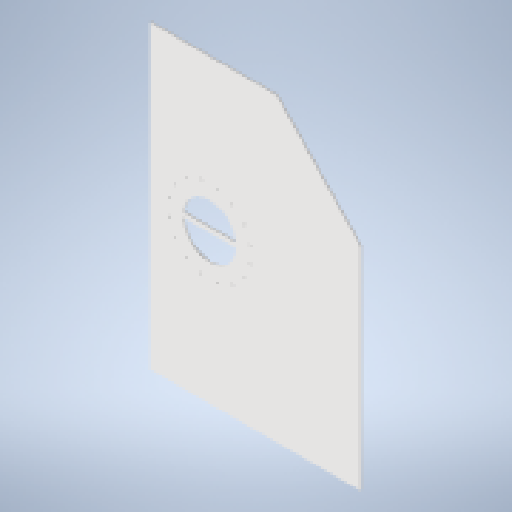
# Autodesk Inventor part: ДМФ 012 Стенка Корма ПРАВ
Saved by Autodesk Inventor 2024.2 (Build 282272000, 272)
## iProperties
Created: 2023-08-31
Part Number: ДМФ 012 Стенка Корма ПРАВ
Material: Generic
Document SubType Name: Sheet Metal
Designer: admin
Stock Number: ДМФ 010 Стенка_Корма
Density: 1 g/cm^3
Flat Pattern Width: 134 cm
Flat Pattern Length: 191 cm
Flat Pattern Area: 25594 cm^2
Sheet Metal Rule: Default
Sheet Metal Width: 1340,000 mm
Sheet Metal Length: 1910,000 mm
Sheet Metal Area: 2559400,000 mm^2
Appearance: Default
Author: admin
Autodesk Inventor part; units mm, degrees
ref_plane "YZ Plane" through (0, 0, 0) normal (1, 0, 0) x (0, 1, 0)
ref_plane "XZ Plane" through (0, 0, 0) normal (0, 1, 0) x (-1, 0, 0)
ref_plane "XY Plane" through (0, 0, 0) normal (0, 0, 1) x (1, 0, 0)
sketch "Sketch1" plane through (0, 0, 0) normal (0, 0, 1) x (1, 0, 0)
  line L0 (0, 0) -> (0, 1910) construction
  line L1 (424.5155, 1910) -> (-415.4845, 1910)
  line L2 (-415.4845, 1910) -> (-1180, 1150)
  line L3 (-1180, 0) -> (-1180, 1150)
  line L4 (960, 0) -> (960, 1342.8524)
  line L5 (424.5155, 1910) -> (960, 1342.8524)
  circle A0 centre (0, 950) radius 265 construction
  line L6 (960, 0) -> (-1180, 0)
  circle A1 centre (-1701.6377, -269.2167) radius 188.5 construction
  circle A2 centre (-800, 80) radius 55
  circle A3 centre (0, 950) radius 170
  line L7 (0, 1215) -> (0, 1120) construction
  line L8 (-721.2646, 955) -> (721.2646, 955) construction
  line L9 (-169.9265, 955) -> (-174.9265, 955) construction
  line L10 (-174.9265, 960) -> (-174.9265, 950)
  line L11 (-174.9265, 960) -> (-169.7056, 960)
  line L12 (-174.9265, 950) -> (-170, 950)
  line L13 (169.9265, 955) -> (174.9265, 955) construction
  line L14 (174.9265, 960) -> (174.9265, 950)
  line L15 (169.7056, 960) -> (174.9265, 960)
  line L16 (174.9265, 950) -> (170, 950)
  line L17 (-174.9265, 970) -> (174.9265, 970)
  line L18 (174.9265, 970) -> (174.9265, 940)
  line L19 (174.9265, 940) -> (-174.9265, 940)
  line L20 (-174.9265, 940) -> (-174.9265, 970)
  arc A4 (-2.4999, 780.0184) -> (2.4999, 780.0184) centre (0, 780) ccw
  arc A5 (2.4999, 1119.9816) -> (-2.4999, 1119.9816) centre (0, 1120) ccw
  point P0 (0, 955)
  point P1 (-169.7056, 940)
  point P2 (169.7056, 940)
  point P3 (168.8194, 970)
  point P4 (-168.8194, 970)
  dimension "d52" = 530
  dimension "d72" = 340
  dimension "d1" = 840
  dimension "d3" = 1150
  dimension "d12" = 1180
  dimension "d13" = 950
  dimension "d14" = 110
  dimension "d15" = 1910
  dimension "d17" = -521.6377
  dimension "d18" = 377
  dimension "d19" = -269.2167
  dimension "d34" = 380
  dimension "d35" = 80
  dimension "d37" = 2140
  dimension "d53" = 5
  dimension "d54" = 10
  dimension "d55" = 30
  dimension "d67" = 5
  dimension "d68" = 5
  dimension "d69" = 780
  dimension "d71" = 1078
  constraints: 42 end point, 10 point on line, 8 horizontal, 6 midpoint, 5 vertical, 4 centre point, 4 point on circle, 2 coincident, 2 equal length, 2 parallel, 1 perpendicular, 1 vertical alignment, 16 other
  measures "d1" distance of L1.start L1.end
  measures "d3" distance of L3.start L2.end
  measures "d12" distance from line of L3 point (0, 950)
  measures "d13" distance from line of L6 point (0, 950)
  measures "d14" diameter of A2
  measures "d15" vertical distance of L3.start L1.end
  measures "d17" distance from line of L3 A1.centre
  measures "d18" diameter of A1
  measures "d19" distance from line of A1.centre L6
  measures "d34" distance from line of A2.centre L3
  measures "d35" distance from line of A2.centre L6
  measures "d37" distance between parallel lines of L4 L3
  measures "d53" distance of L9.end L9.start
  measures "d54" distance of L10.start L10.end
  measures "d55" distance between parallel lines of L19 L17
  measures "d67" diameter of A4
  measures "d68" diameter of A5
  measures "d69" distance of L1.start L4.end
  measures "d71" distance of L1.end L2.end
extrude "Extrusion1" add sketch "Sketch1" along normal blind 10 contours L5 L4 L6 L3 L2 L1 | A3 L19 L17 | L16 L18 L19 A3 | A3 L15 L14 L16 | A3 L17 L18 L15 | L19 L20 L12 A3 | A3 L11 L20 L17 | L12 L10 L11 A3
fillet "Fillet1" radius 10 4 edges at (-168.8194, 970, 5) (-169.7056, 940, 5) (168.8194, 970, 5) (169.7056, 940, 5)
sketch "Sketch4" plane through (0, 0, 0) normal (0, 0, 1) x (1, 0, 0)
  circle A0 centre (-51.6989, 1209.9081) radius 6.5
  arc A1 (-2.4999, 1119.9816) -> (-166.985, 981.875) centre (0, 950) ccw projected
  line L0 (0, 950) -> (0, 1196.7062) construction
  line L1 (-51.6989, 1209.9081) -> (0, 950) construction
  point P0 (0, 0)
  point P1 (-5, 1149.9375)
  dimension "d59" = 265
  dimension "d60" = 13
  dimension "d61" = 11.25
  constraints: 4 end point, 1 centre point, 1 vertical
  measures "d59" distance of L0.start L1.start
  measures "d60" diameter of A0
  measures "d61" angle of L1 L0
extrude "Extrusion4" cut sketch "Sketch4" along normal blind 10
pattern_circular "Circular Pattern3" count 16 over 360 about axis through (0, 950, 0) along (0, 0, 1) of "Extrusion4"
sketch "Sketch5" plane through (0, 0, 10) normal (0, 0, 1) x (1, 0, 0)
  circle A0 centre (51.6989, 1209.9081) radius 6.5 projected
  circle A1 centre (147.2261, 1170.3394) radius 6.5 projected
  circle A2 centre (220.3394, 1097.2261) radius 6.5 projected
  circle A3 centre (259.9081, 1001.6989) radius 6.5 projected
  circle A4 centre (259.9081, 898.3011) radius 6.5 projected
  circle A5 centre (220.3394, 802.7739) radius 6.5 projected
  circle A6 centre (147.2261, 729.6606) radius 6.5 projected
  circle A7 centre (51.6989, 690.0919) radius 6.5 projected
  circle A8 centre (-51.6989, 690.0919) radius 6.5 projected
  circle A9 centre (-147.2261, 729.6606) radius 6.5 projected
  circle A10 centre (-220.3394, 802.7739) radius 6.5 projected
  circle A11 centre (-259.9081, 898.3011) radius 6.5 projected
  circle A12 centre (-259.9081, 1001.6989) radius 6.5 projected
  circle A13 centre (-220.3394, 1097.2261) radius 6.5 projected
  circle A14 centre (-147.2261, 1170.3394) radius 6.5 projected
  circle A15 centre (-51.6989, 1209.9081) radius 6.5 projected
  line L0 (960, 1342.8524) -> (424.5155, 1910) projected
  line L1 (424.5155, 1910) -> (-415.4845, 1910) projected
  line L2 (-415.4845, 1910) -> (-1180, 1150) projected
  line L3 (-1180, 1150) -> (-1180, 0) projected
  line L4 (-1180, 0) -> (960, 0) projected
  line L5 (960, 0) -> (960, 1342.8524) projected
  arc A16 (2.4999, 780.0184) -> (168.6666, 928.75) centre (0, 950) ccw projected
  arc A17 (-2.4999, 780.0184) -> (2.4999, 780.0184) centre (0, 780) ccw projected
  arc A18 (-168.6666, 928.75) -> (-2.4999, 780.0184) centre (0, 950) ccw projected
  arc A19 (-158.7451, 940) -> (-168.6666, 928.75) centre (-158.7451, 930) ccw projected
  line L6 (-158.7451, 940) -> (158.7451, 940) projected
  arc A20 (168.6666, 928.75) -> (158.7451, 940) centre (158.7451, 930) ccw projected
  circle A21 centre (-800, 80) radius 55 projected
  line L7 (157.1623, 970) -> (-157.1623, 970) projected
  arc A22 (-166.985, 981.875) -> (-157.1623, 970) centre (-157.1623, 980) ccw projected
  arc A23 (-2.4999, 1119.9816) -> (-166.985, 981.875) centre (0, 950) ccw projected
  arc A24 (2.4999, 1119.9816) -> (-2.4999, 1119.9816) centre (0, 1120) ccw projected
  arc A25 (166.985, 981.875) -> (2.4999, 1119.9816) centre (0, 950) ccw projected
  arc A26 (157.1623, 970) -> (166.985, 981.875) centre (157.1623, 980) ccw projected
  line L8 (-380, 0) -> (-380, 1910)
  point P0 (0, 0)
  dimension "d73" = 1340
  constraints: 2 end point, 2 point on line, 1 perpendicular
  measures "d73" distance between parallel lines of L5 L8
extrude "Extrusion5" cut sketch "Sketch5" against normal through all contours L8 L4 L3 L2 L1
body "Solid1"
